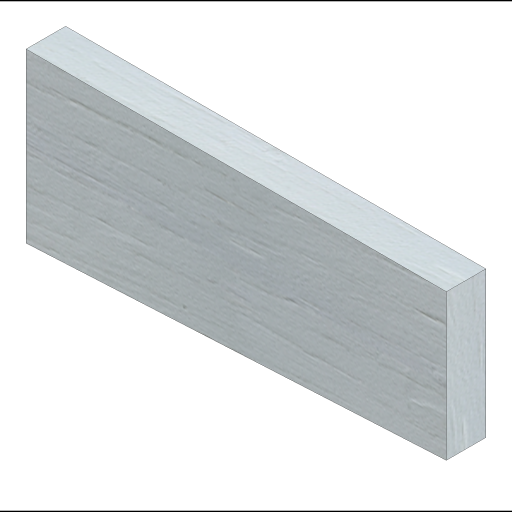
# Autodesk Inventor part: Antitorque Outlet Support
Saved by Autodesk Inventor 2023 (Build 270158000, 158)
## iProperties
Created: 2023-01-26
Part Number: Antitorque Outlet Support
Material: Wood (Oak)
Document SubType Name: Modeling
Designer: kamer
Density: 0.76 g/cm^3
Appearance: Wood - Painted White
Author: kamer
Autodesk Inventor part; units mm, degrees
ref_plane "YZ Plane" through (0, 0, 0) normal (1, 0, 0) x (0, 1, 0)
ref_plane "XZ Plane" through (0, 0, 0) normal (0, 1, 0) x (-1, 0, 0)
ref_plane "XY Plane" through (0, 0, 0) normal (0, 0, 1) x (1, 0, 0)
sketch "Sketch1" plane through (0, 0, 0) normal (0, 0, 1) x (1, 0, 0)
  line L0 (0, 0) -> (969.3217, 0)
  line L1 (969.3217, 0) -> (969.3217, 50.8)
  line L2 (969.3217, 50.8) -> (0, 50.8)
  line L3 (0, 50.8) -> (0, 0)
  line L4 (0, 0) -> (969.3217, 50.8)
  line L5 (127, 0) -> (127, 50.8)
  point P0 (0, 25.4)
  point P1 (127, 6.6558)
  dimension "d0" = 3
  dimension "d4" = 50.8
  dimension "d5" = 127
  constraints: 12 end point, 2 parallel, 2 perpendicular, 2 point on line, 1 horizontal, 1 midpoint
  measures "d0" angle of L0 L4
  measures "d4" distance of L0.end L1.end
  measures "d5" distance from line of point (0, 25.4) L5
extrude "Extrusion2" add sketch "Sketch1" along normal blind 11.938 contours L3 L2 L5 L4
body "Solid2"
